esp32_7_seg_v3 (Autodesk Fusion 360 design; units mm, degrees)
Autodesk Fusion 360 part; units mm, degrees
sketch "profile" plane through (0, 0, 0) normal (1, 0, 0) x (0, 0, -1)
  line L0 (0, 0) -> (-26, 0)
  line L1 (-26, 0) -> (-26, 3)
  line L2 (-26, 3) -> (-20.0762, 18.9227)
  line L3 (0, 0) -> (0, 3)
  line L4 (-0.6304, 4.4574) -> (-16.8321, 19.6828)
  arc A0 (-16.8321, 19.6828) -> (-20.0762, 18.9227) centre (-18.2017, 18.2254) ccw
  arc A1 (0, 3) -> (-0.6304, 4.4574) centre (-2, 3) ccw
  point P0 (-19.0263, 21.7448)
  dimension "d1" = 26
  dimension "d2" = 3
  dimension "d3" = 20
  dimension "d4" = 2
  dimension "d5" = 2
  constraint coincident L0.start L3.start
  constraint horizontal L0
  constraint perpendicular L0 L1
  constraint perpendicular L0 L3
  constraint coincident P0 L2
  constraint coincident P0 L4
  constraint tangent L2 A0
  constraint tangent L4 A0
  constraint tangent L3 A1
  constraint tangent L4 A1
  constraint equal L1 L3
  measures "d1" distance of L0.start L0.end
  measures "d2" distance of L0.end L1.end
  measures "d3" distance of L1.end P0
  measures "d4" radius of A0
  measures "d5" radius of A1
extrude "Extrude1" add sketch "profile" along normal blind 85 makes body 1
shell "Shell1" thickness 1 outward yes removed faces 0 bodies 1
sketch "FACE" plane through (0, 2.7812, -2.6136) normal (0, 0.728723, -0.684809) x (-1, 0, 0)
  line L0 (1, 3.5119) -> (1, 25.7449)
  line L1 (1, 25.7449) -> (-86, 25.7449)
  line L2 (-86, 25.7449) -> (-86, 3.5119)
  line L3 (-86, 3.5119) -> (1, 3.5119)
  line L4 (-74, 22.6284) -> (-11, 22.6284)
  line L5 (-11, 22.6284) -> (-11, 6.6284)
  line L6 (-11, 6.6284) -> (-74, 6.6284)
  line L7 (-74, 6.6284) -> (-74, 22.6284)
  line L8 (-86, 14.6284) -> (-74, 14.6284)
  line L9 (-11, 14.6284) -> (1, 14.6284)
  line L10 (-42.5, 22.6284) -> (-42.5, 25.7449)
  line L11 (-42.5, 6.6284) -> (-42.5, 3.5119)
  dimension "d10" = 63
  dimension "d11" = 16
  constraint horizontal L4
  constraint vertical L5
  constraint horizontal L6
  constraint vertical L7
  constraint midpoint L2 L8.start
  constraint midpoint L7 L8.end
  constraint midpoint L5 L9.start
  constraint midpoint L0 L9.end
  constraint midpoint L4 L10.start
  constraint midpoint L1 L10.end
  constraint midpoint L6 L11.start
  constraint midpoint L3 L11.end
  constraint equal L8 L9
  constraint equal L10 L11
  measures "d10" distance of L4.start L4.end
  measures "d11" distance of L4.start L6.end
extrude "Extrude2" cut sketch "FACE" against normal blind 9 contours L4 L5 L6 L7 bodies 1
sketch "Port" plane through (86, 0, 0) normal (1, 0, 0) x (0, 0, -1)
  line L0 (1, -1) -> (1, 3)
  arc A0 (1, 3) -> (0.0544, 5.1862) centre (-2, 3) ccw
  line L1 (0.0544, 5.1862) -> (-16.1473, 20.4115)
  arc A1 (-16.1473, 20.4115) -> (-21.0134, 19.2714) centre (-18.2017, 18.2254) ccw
  line L2 (-21.0134, 19.2714) -> (-27, 3.18)
  line L3 (-27, 3.18) -> (-27, -1)
  line L4 (-27, -1) -> (1, -1)
  line L5 (-13, -1) -> (-13, 0)
  line L6 (-13, 0) -> (-8, 0)
  line L7 (-8, 0) -> (-8, 4)
  line L8 (-8, 4) -> (-18, 4)
  line L9 (-18, 4) -> (-18, 0)
  line L10 (-18, 0) -> (-13, 0)
  constraint midpoint L4 L5.start
  constraint perpendicular L4 L5
  constraint perpendicular L5 L6
  constraint perpendicular L4 L7
  constraint perpendicular L7 L8
  constraint perpendicular L8 L9
  constraint perpendicular L5 L10
extrude "Extrude3" cut sketch "Port" against normal blind 3 contours L6 L7 L8 L9 L10 bodies 1
sketch "Cutout" plane through (-1, 0, 0) normal (-1, 0, 0) x (0, 0, 1)
  line L0 (-1, 3) -> (-1, -1)
  line L1 (-1, -1) -> (27, -1)
  line L2 (27, -1) -> (27, 3.18)
  line L3 (27, 3.18) -> (21.0134, 19.2714)
  arc A0 (21.0134, 19.2714) -> (16.1473, 20.4115) centre (18.2017, 18.2254) ccw
  line L4 (16.1473, 20.4115) -> (-0.0544, 5.1862)
  arc A1 (-0.0544, 5.1862) -> (-1, 3) centre (2, 3) ccw
  line L5 (13, -1) -> (13, 0)
  line L6 (-1, -1) -> (-1, 0)
  line L7 (27, -1) -> (27, 0)
  line L8 (27, 0) -> (24, 0)
  line L9 (-1, 0) -> (2, 0)
  line L10 (2, 0) -> (2.25, 0)
  line L11 (24, 0) -> (23.75, 0)
  line L12 (23.75, 0) -> (2.25, 0)
  line L13 (2, 0) -> (2, -1)
  line L14 (24, 0) -> (24, -1)
  line L15 (2.25, 0) -> (2.25, -1)
  line L16 (23.75, 0) -> (23.75, -1)
  line L17 (2.25, 0) -> (2.25, 1)
  line L18 (2.25, 1) -> (0.25, 1)
  line L19 (0.25, 1) -> (0.25, 0)
  line L20 (24, 1) -> (25.75, 1)
  line L21 (25.75, 1) -> (25.75, 0)
  line L22 (2.25, 1) -> (24, 1)
  line L23 (23.75, 0) -> (23.75, -1)
  line L24 (2.25, 0) -> (2.25, -1)
  line L25 (0.25, 1) -> (0, 1)
  line L26 (0, 1) -> (0, 0)
  line L27 (25.75, 1) -> (26, 1)
  line L28 (26, 1) -> (26, 0)
  line L29 (26, 0.5) -> (27, 0.5)
  line L30 (0, 0.5) -> (-1, 0.5)
  dimension "d16" = 0.25
  dimension "d17" = 0.25
  dimension "d18" = 3
  dimension "d19" = 3
  dimension "d20" = 1
  dimension "d21" = 2
  dimension "d22" = 3
  dimension "d23" = 3
  dimension "d24" = 0
  constraint midpoint L1 L5.start
  constraint perpendicular L1 L5
  constraint coincident L0.end L1.start
  constraint coincident L0 L6.end
  constraint coincident L1.end L2.start
  constraint coincident L2 L7.end
  constraint perpendicular L2 L8
  constraint perpendicular L6 L9
  constraint horizontal L10
  constraint parallel L8 L11
  constraint parallel L10 L12
  constraint equal L10 L11
  constraint equal L8 L9
  constraint coincident L1 L13.end
  constraint perpendicular L1 L13
  constraint coincident L1 L14.end
  constraint perpendicular L1 L14
  constraint coincident L1 L15.end
  constraint perpendicular L1 L15
  constraint coincident L1 L16.end
  constraint perpendicular L1 L16
  constraint perpendicular L10 L17
  constraint perpendicular L17 L18
  constraint coincident L9 L19.end
  constraint perpendicular L9 L19
  constraint perpendicular L17 L20
  constraint coincident L8 L21.end
  constraint perpendicular L8 L21
  constraint perpendicular L21 L22
  constraint perpendicular L19 L25
  constraint coincident L26.end origin
  constraint perpendicular L9 L26
  constraint perpendicular L21 L27
  constraint coincident L8 L28.end
  constraint perpendicular L8 L28
  constraint equal L25 L27
  constraint midpoint L28 L29.start
  constraint coincident L2 L29.end
  constraint perpendicular L2 L29
  constraint midpoint L26 L30.start
  constraint coincident L0 L30.end
  constraint perpendicular L0 L30
  constraint equal L29 L30
  measures "d16" distance of L9.end L10.end
  measures "d17" distance of L8.end L11.end
  measures "d18" distance of L7.end L8.end
  measures "d19" distance of L6.end L9.end
  measures "d20" distance of L5.start L5.end
  measures "d21" distance of L17.end L18.end
  measures "d22" distance of L6.end L9.end
  measures "d23" distance of L7.end L8.end
  measures "d24" distance of L20 L22
extrude "Extrude4" cut sketch "Cutout" against normal blind 20.25 contours L9 L19 L25 L26 | L1 L10 L13 L15 L24 | L9 L10 L17 L18 L19 | L1 L5 L12 L15 L24 | L8 L11 L12 L17 L20 L21 L22 | L1 L5 L12 L16 L23 | L8 L21 L27 L28 | L1 L11 L14 L16 L23 bodies 1
extrude "Extrude5" add sketch "Cutout" against normal blind 20 separate body contours L9 L10 L17 L18 L19 | L1 L5 L12 L15 L24 | L8 L11 L12 L17 L20 L21 L22 | L1 L5 L12 L16 L23 makes body 2
extrude "Extrude6" add sketch "Cutout" against normal blind 21 contours L9 L10 L17 L18 L19 | L8 L11 L12 L17 L20 L21 L22 bodies 2
extrude "Extrude7" add 1 faces at (20, 0.6667, 8.75) along direction (1, 0, 0) blind 1 on bodies 2 bodies 2
named bodies: "Body", "Back"
